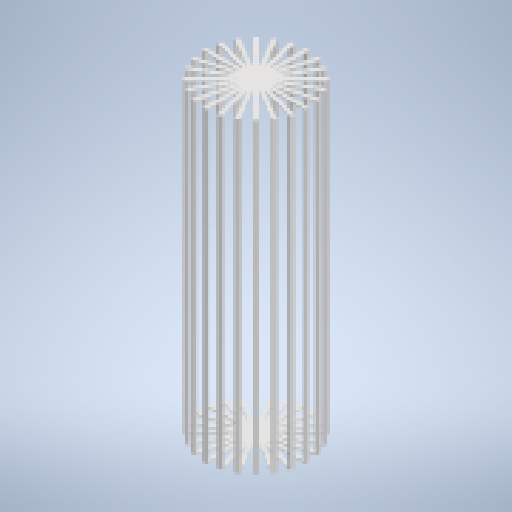
# Autodesk Inventor part: Liga recolector
Saved by Autodesk Inventor 2024 (Build 280153000, 153)
## iProperties
Created: 2023-10-30
Part Number: Liga recolector
Material: Genérico
Document SubType Name: Modeling
Designer: ismae
Density: 1 g/cm^3
Appearance: Valor por defecto
Author: ismae
Autodesk Inventor part; units mm, degrees
ref_plane "YZ Plane" through (0, 0, 0) normal (1, 0, 0) x (0, 1, 0)
ref_plane "XZ Plane" through (0, 0, 0) normal (0, 1, 0) x (-1, 0, 0)
sketch "Boceto1" plane through (0, 0, 0) normal (0, 1, 0) x (-1, 0, 0)
  circle A0 centre (0, 0) radius 38.481
  line L0 (1.5, 38.4518) -> (-1.5, 38.4518)
  line L1 (-1.5, 38.4518) -> (-1.5, -38.4518)
  line L2 (-1.5, -38.4518) -> (1.5, -38.4518)
  line L3 (1.5, -38.4518) -> (1.5, 38.4518)
  line L4 (1.5, 38.4518) -> (-1.5, -38.4518) construction
  line L5 (-1.5, 38.4518) -> (1.5, -38.4518) construction
  line L6 (-11.4009, 36.7533) -> (8.5032, -37.5298)
  line L7 (11.4009, -36.7533) -> (-8.5032, 37.5298)
  circle A1 centre (0, 0) radius 38.481
  line L8 (-20.5249, 32.5502) -> (17.9268, -34.0502)
  line L9 (20.5249, -32.5502) -> (-17.9268, 34.0502)
  circle A2 centre (0, 0) radius 38.481
  line L10 (-28.2502, 26.1288) -> (26.1288, -28.2502)
  line L11 (28.2502, -26.1288) -> (-26.1288, 28.2502)
  circle A3 centre (0, 0) radius 38.481
  line L12 (-34.0502, 17.9268) -> (32.5502, -20.5249)
  line L13 (34.0502, -17.9268) -> (-32.5502, 20.5249)
  circle A4 centre (0, 0) radius 38.481
  line L14 (-37.5298, 8.5032) -> (36.7533, -11.4009)
  line L15 (37.5298, -8.5032) -> (-36.7533, 11.4009)
  circle A5 centre (0, 0) radius 38.481
  line L16 (-38.4518, -1.5) -> (38.4518, -1.5)
  line L17 (38.4518, 1.5) -> (-38.4518, 1.5)
  circle A6 centre (0, 0) radius 38.481
  line L18 (-36.7533, -11.4009) -> (37.5298, 8.5032)
  line L19 (36.7533, 11.4009) -> (-37.5298, -8.5032)
  circle A7 centre (0, 0) radius 38.481
  line L20 (-32.5502, -20.5249) -> (34.0502, 17.9268)
  line L21 (32.5502, 20.5249) -> (-34.0502, -17.9268)
  circle A8 centre (0, 0) radius 38.481
  line L22 (-26.1288, -28.2502) -> (28.2502, 26.1288)
  line L23 (26.1288, 28.2502) -> (-28.2502, -26.1288)
  circle A9 centre (0, 0) radius 38.481
  line L24 (-17.9268, -34.0502) -> (20.5249, 32.5502)
  line L25 (17.9268, 34.0502) -> (-20.5249, -32.5502)
  circle A10 centre (0, 0) radius 38.481
  line L26 (-8.5032, -37.5298) -> (11.4009, 36.7533)
  line L27 (8.5032, 37.5298) -> (-11.4009, -36.7533)
  circle A11 centre (0, 0) radius 38.481
  line L28 (1.5, -38.4518) -> (1.5, 38.4518)
  line L29 (-1.5, 38.4518) -> (-1.5, -38.4518)
  circle A12 centre (0, 0) radius 38.481
  line L30 (11.4009, -36.7533) -> (-8.5032, 37.5298)
  line L31 (-11.4009, 36.7533) -> (8.5032, -37.5298)
  circle A13 centre (0, 0) radius 38.481
  line L32 (20.5249, -32.5502) -> (-17.9268, 34.0502)
  line L33 (-20.5249, 32.5502) -> (17.9268, -34.0502)
  circle A14 centre (0, 0) radius 38.481
  line L34 (28.2502, -26.1288) -> (-26.1288, 28.2502)
  line L35 (-28.2502, 26.1288) -> (26.1288, -28.2502)
  circle A15 centre (0, 0) radius 38.481
  line L36 (34.0502, -17.9268) -> (-32.5502, 20.5249)
  line L37 (-34.0502, 17.9268) -> (32.5502, -20.5249)
  circle A16 centre (0, 0) radius 38.481
  line L38 (37.5298, -8.5032) -> (-36.7533, 11.4009)
  line L39 (-37.5298, 8.5032) -> (36.7533, -11.4009)
  circle A17 centre (0, 0) radius 38.481
  line L40 (38.4518, 1.5) -> (-38.4518, 1.5)
  line L41 (-38.4518, -1.5) -> (38.4518, -1.5)
  circle A18 centre (0, 0) radius 38.481
  line L42 (36.7533, 11.4009) -> (-37.5298, -8.5032)
  line L43 (-36.7533, -11.4009) -> (37.5298, 8.5032)
  circle A19 centre (0, 0) radius 38.481
  line L44 (32.5502, 20.5249) -> (-34.0502, -17.9268)
  line L45 (-32.5502, -20.5249) -> (34.0502, 17.9268)
  circle A20 centre (0, 0) radius 38.481
  line L46 (26.1288, 28.2502) -> (-28.2502, -26.1288)
  line L47 (-26.1288, -28.2502) -> (28.2502, 26.1288)
  circle A21 centre (0, 0) radius 38.481
  line L48 (17.9268, 34.0502) -> (-20.5249, -32.5502)
  line L49 (-17.9268, -34.0502) -> (20.5249, 32.5502)
  circle A22 centre (0, 0) radius 38.481
  line L50 (8.5032, 37.5298) -> (-11.4009, -36.7533)
  line L51 (-8.5032, -37.5298) -> (11.4009, 36.7533)
  circle A23 centre (0, 0) radius 38.481
  circle A24 centre (0, 0) radius 36.8218
  point P0 (4.3978, -10.6172)
  point P1 (6.9959, -9.1172)
  point P2 (9.1172, -6.9959)
  point P3 (10.6172, -4.3978)
  point P4 (11.3936, -1.5)
  point P5 (11.3936, 1.5)
  point P6 (10.6172, 4.3978)
  point P7 (34.0502, 17.9268)
  point P8 (9.1172, 6.9959)
  point P9 (6.9959, 9.1172)
  point P10 (4.3978, 10.6172)
  point P11 (1.5, 11.3936)
  point P12 (-1.5, 11.3936)
  point P13 (-4.3978, 10.6172)
  point P14 (-6.9959, 9.1172)
  point P15 (-9.1172, 6.9959)
  point P16 (-11.3936, 1.5)
  point P17 (-11.3936, -1.5)
  point P18 (-10.6172, -4.3978)
  point P19 (-34.0502, -17.9268)
  point P20 (-9.1172, -6.9959)
  point P21 (-6.9959, -9.1172)
  point P22 (-4.3978, -10.6172)
  point P23 (-1.5, -11.3936)
  point P24 (1.5, -11.3936)
  point P25 (-10.6172, 4.3978)
  dimension "d0" = 76.962
  dimension "d1" = 3
  dimension "d4" = 360
  constraints: 104 end point, 4 coincident, 2 midpoint, 2 parallel, 1 centre point, 1 horizontal, 1 perpendicular, 263 other
  measures "d1" distance of L2.end L1.end
extrude "Extrusión1" add sketch "Boceto1" along normal blind 230.124 contours A0 L16 A24 L17 | L18 A24 L19 A0 | A24 L16 L15 L18 L17 | A0 L14 A24 L15 | L18 L17 L20 L19 A24 | L18 L15 L20 L17 | A24 L14 L13 L16 L15 | L16 L13 L18 L15 | L20 A24 L21 A0 | L20 L15 L22 L17 | L17 L22 L19 L20 | L18 L13 L20 L15 | A0 L12 A24 L13 | L16 L11 L18 L13 | L13 L14 L11 L16 | L20 L19 L22 L21 A24 | L22 L15 L24 L17 | L17 L24 L19 L22 | L20 L13 L22 L15 | L18 L11 L20 L13 | A24 L12 L11 L14 L13 | L16 L9 L18 L11 | L11 L14 L9 L16 | L22 A24 L23 A0 | L19 L24 L21 L22 | L24 L15 L26 L17 | L17 L26 L19 L24 | L22 L13 L24 L15 | L20 L11 L22 L13 | L18 L9 L20 L11 | A0 L10 A24 L11 | L11 L12 L9 L14 | L16 L7 L18 L9 | L9 L14 L7 L16 | L22 L21 L24 L23 A24 | L19 L26 L21 L24 | L26 L15 L3 L17 | L17 L3 L19 L26 | L24 L13 L26 L15 | L22 L11 L24 L13 | L20 L9 L22 L11 | L18 L7 L20 L9 | A24 L10 L9 L12 L11 | L9 L12 L7 L14 | L16 L3 L18 L7 | L7 L14 L3 L16 | L24 A24 L25 A0 | L21 L26 L23 L24 | L19 L3 L21 L26 | L17 L7 L19 L3 | L3 L15 L7 L17 | L26 L13 L3 L15 | L24 L11 L26 L13 | L22 L9 L24 L11 | L20 L7 L22 L9 | L18 L3 L20 L7 | A0 L8 A24 L9 | L9 L10 L7 L12 | L7 L12 L3 L14 | L16 L26 L18 L3 | L3 L14 L26 L16 | L24 L23 L26 L25 A24 | L21 L3 L23 L26 | L19 L7 L21 L3 | L3 L13 L7 L15 | L17 L9 L19 L7 | L7 L15 L9 L17 | L26 L11 L3 L13 | L24 L9 L26 L11 | L22 L7 L24 L9 | L20 L3 L22 L7 | L18 L26 L20 L3 | A24 L8 L7 L10 L9 | L7 L10 L3 L12 | L3 L12 L26 L14 | L26 L14 L24 L16 | L16 L24 L18 L26 | L26 A24 L27 A0 | L23 L3 L25 L26 | L21 L7 L23 L3 | L19 L9 L21 L7 | L3 L11 L7 L13 | L7 L13 L9 L15 | L17 L11 L19 L9 | L9 L15 L11 L17 | L26 L9 L3 L11 | L24 L7 L26 L9 | L22 L3 L24 L7 | L20 L26 L22 L3 | L18 L24 L20 L26 | A0 L6 A24 L7 | L7 L8 L3 L10 | L3 L10 L26 L12 | L26 L12 L24 L14 | L24 L14 L22 L16 | L16 L22 L18 L24 | L26 L25 L3 L27 A24 | L23 L7 L25 L3 | L21 L9 L23 L7 | L19 L11 L21 L9 | L3 L9 L7 L11 | L7 L11 L9 L13 | L9 L13 L11 L15 | L17 L13 L19 L11 | L11 L15 L13 L17 | L26 L7 L3 L9 | L24 L3 L26 L7 | L22 L26 L24 L3 | L20 L24 L22 L26 | L18 L22 L20 L24 | A24 L6 L3 L8 L7 | L3 L8 L26 L10 | L26 L10 L24 L12 | L24 L12 L22 L14 | L22 L14 L20 L16 | L16 L20 L18 L22 | L3 A24 L1 L0 | L25 L7 L27 L3 | L23 L9 L25 L7 | L21 L11 L23 L9 | L19 L13 L21 L11 | L3 L7 L9 | L7 L9 L11 | L9 L11 L13 | L11 L13 L15 | L17 L15 L19 L13 | L13 L15 L17 | L26 L3 L7 | L24 L26 L3 | L22 L24 L26 | L20 L22 L24 | L18 L20 L22 | L2 L1 A24 L3 | L3 L6 L26 L8 | L26 L8 L24 L10 | L24 L10 L22 L12 | L22 L12 L20 L14 | L20 L14 L18 L16 | L16 L18 L20 | L3 L27 L7 L1 A24 | L25 L9 L27 L7 | L23 L11 L25 L9 | L21 L13 L23 L11 | L19 L15 L21 L13 | L3 L26 L24 L22 L20 L18 L16 L14 L12 L10 L8 L6 L1 L27 L25 L23 L21 L19 L17 L15 L13 L11 L9 L7 | L17 L19 L15 | A24 L1 L26 L6 L3 | L26 L6 L24 L8 | L24 L8 L22 L10 | L22 L10 L20 L12 | L20 L12 L18 L14 | L18 L14 L16 | L7 A24 L6 A0 | L27 L9 L1 L7 | L25 L11 L27 L9 | L23 L13 L25 L11 | L21 L15 L23 L13 | L19 L17 L21 L15 | L19 L21 L17 | A0 L27 A24 L26 | L26 L1 L24 L6 | L24 L6 L22 L8 | L22 L8 L20 L10 | L20 L10 L18 L12 | L18 L12 L16 L14 | L16 L12 L14 | L7 L1 L9 L6 A24 | L27 L11 L1 L9 | L25 L13 L27 L11 | L23 L15 L25 L13 | L21 L17 L23 L15 | L21 L19 L23 L17 | L21 L23 L19 | A24 L27 L24 L1 L26 | L24 L1 L22 L6 | L22 L6 L20 L8 | L20 L8 L18 L10 | L18 L10 L16 L12 | L14 L10 L12 | L12 L16 L10 L14 | L9 A24 L8 A0 | L1 L11 L6 L9 | L27 L13 L1 L11 | L25 L15 L27 L13 | L23 L17 L25 L15 | L23 L19 L25 L17 | L23 L21 L25 L19 | L23 L25 L21 | A0 L25 A24 L24 | L24 L27 L22 L1 | L22 L1 L20 L6 | L20 L6 L18 L8 | L18 L8 L16 L10 | L12 L8 L10 | L10 L14 L8 L12 | L10 L16 L8 L14 | L9 L6 L11 L8 A24 | L1 L13 L6 L11 | L27 L15 L1 L13 | L25 L17 L27 L15 | L25 L19 L27 L17 | L25 L21 L27 L19 | L25 L23 L27 L21 | L25 L27 L23 | A24 L25 L22 L27 L24 | L22 L27 L20 L1 | L20 L1 L18 L6 | L18 L6 L16 L8 | L10 L6 L8 | L8 L12 L6 L10 | L8 L14 L6 L12 | L8 L16 L6 L14 | L11 A24 L10 A0 | L6 L13 L8 L11 | L1 L15 L6 L13 | L27 L17 L1 L15 | L27 L19 L1 L17 | L27 L21 L1 L19 | L27 L23 L1 L21 | L27 L25 L1 L23 | L27 L1 L25 | A0 L23 A24 L22 | L22 L25 L20 L27 | L20 L27 L18 L1 | L18 L1 L16 L6 | L8 L1 L6 | L6 L10 L1 L8 | L6 L12 L1 L10 | L6 L14 L1 L12 | L6 L16 L1 L14 | L11 L8 L13 L10 A24 | L6 L15 L8 L13 | L1 L17 L6 L15 | L1 L19 L6 L17 | L1 L21 L6 L19 | L1 L23 L6 L21 | L1 L25 L6 L23 | L1 L27 L6 L25 | L1 L6 L27 | A24 L23 L20 L25 L22 | L20 L25 L18 L27 | L18 L27 L16 L1 | L1 L8 L27 L6 | L1 L10 L27 L8 | L1 L12 L27 L10 | L1 L14 L27 L12 | L1 L16 L27 L14 | L13 A24 L12 A0 | L8 L15 L10 L13 | L6 L17 L8 L15 | L6 L19 L8 L17 | L6 L21 L8 L19 | L6 L23 L8 L21 | L6 L25 L8 L23 | L6 L27 L8 L25 | A0 L21 A24 L20 | L20 L23 L18 L25 | L18 L25 L16 L27 | L27 L10 L25 L8 | L27 L12 L25 L10 | L27 L14 L25 L12 | L27 L16 L25 L14 | L13 L10 L15 L12 A24 | L8 L17 L10 L15 | L8 L19 L10 L17 | L8 L21 L10 L19 | L8 L23 L10 L21 | L8 L25 L10 L23 | A24 L21 L18 L23 L20 | L18 L23 L16 L25 | L25 L12 L23 L10 | L25 L14 L23 L12 | L25 L16 L23 L14 | L15 A24 L14 A0 | L10 L17 L12 L15 | L10 L19 L12 L17 | L10 L21 L12 L19 | L10 L23 L12 L21 | A0 L19 A24 L18 | L18 L21 L16 L23 | L23 L14 L21 L12 | L23 L16 L21 L14 | L15 L12 L17 L14 A24 | L12 L19 L14 L17 | L12 L21 L14 L19 | A24 L19 L16 L21 L18 | L21 L16 L19 L14 | L17 A24 L16 A0 | L14 L19 L16 A24 L17
sketch "Boceto2" plane through (0, 0, 0) normal (0, -1, 0) x (1, 0, 0)
  circle A0 centre (0, 0) radius 43.7891
  constraints: 1 centre point, 1 coincident
ref_plane "Plano de trabajo1" through (0, 115.062, 0) normal (0, -1, 0) x (1, 0, 0)
sketch "Boceto3" plane through (0, 115.062, 0) normal (0, -1, 0) x (1, 0, 0)
  circle A0 centre (0, 0) radius 37.0606
  constraints: 1 centre point, 1 coincident
extrude "Extrusión2" cut sketch "Boceto3" along normal mid plane 228.5365
